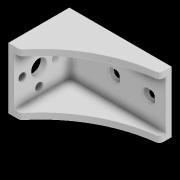
# Autodesk Inventor part: sujetador del motor
Saved by Autodesk Inventor 2020 (Build 240168000, 168)
## iProperties
Created: 2021-11-22
Part Number: sujetador del motor
Material: Generic
Document SubType Name: Modeling
Designer: juan
Density: 1 g/cm^3
Appearance: Default
Author: juan
Autodesk Inventor part; units mm, degrees
ref_plane "YZ Plane" through (0, 0, 0) normal (1, 0, 0) x (0, 1, 0)
ref_plane "XZ Plane" through (0, 0, 0) normal (0, 1, 0) x (-1, 0, 0)
ref_plane "XY Plane" through (0, 0, 0) normal (0, 0, 1) x (1, 0, 0)
sketch "Sketch1" plane through (0, 0, 0) normal (0, 0, 1) x (1, 0, 0)
  line L0 (0, 0) -> (52, 0)
  line L1 (52, 0) -> (52, 31)
  line L2 (52, 31) -> (0, 31)
  line L3 (0, 31) -> (0, 0)
  line L4 (24.7, 18.5) -> (26.7, 18.5)
  line L5 (28.7, 16.5) -> (28.7, 14.5)
  line L6 (26.7, 12.5) -> (24.7, 12.5)
  line L7 (22.7, 14.5) -> (22.7, 16.5)
  arc A0 (22.7, 14.5) -> (24.7, 12.5) centre (24.7, 14.5) ccw
  arc A1 (24.7, 18.5) -> (22.7, 16.5) centre (24.7, 16.5) ccw
  arc A2 (28.7, 16.5) -> (26.7, 18.5) centre (26.7, 16.5) ccw
  arc A3 (26.7, 12.5) -> (28.7, 14.5) centre (26.7, 14.5) ccw
  line L8 (42.542, 18.5) -> (44.542, 18.5)
  line L9 (46.542, 16.5) -> (46.542, 14.5)
  line L10 (44.542, 12.5) -> (42.542, 12.5)
  line L11 (40.542, 14.5) -> (40.542, 16.5)
  arc A4 (40.542, 14.5) -> (42.542, 12.5) centre (42.542, 14.5) ccw
  arc A5 (42.542, 18.5) -> (40.542, 16.5) centre (42.542, 16.5) ccw
  arc A6 (46.542, 16.5) -> (44.542, 18.5) centre (44.542, 16.5) ccw
  arc A7 (44.542, 12.5) -> (46.542, 14.5) centre (44.542, 14.5) ccw
  point P0 (28.7, 12.5)
  point P1 (28.7, 18.5)
  point P2 (22.7, 12.5)
  point P3 (22.7, 15.5)
  point P4 (0, 15.5)
  point P5 (46.542, 12.5)
  point P6 (46.542, 18.5)
  point P7 (40.542, 12.5)
  point P8 (40.542, 15.5)
  point P9 (28.7, 15.5)
  dimension "d0" = 52
  dimension "d1" = 31
  dimension "d2" = 6
  dimension "d3" = 6
  dimension "d4" = 2
  dimension "d5" = 22.7
  dimension "d6" = 6
  dimension "d7" = 6
  dimension "d8" = 2
  dimension "d9" = 5.458
  constraints: 24 end point, 16 point on circle, 16 tangent, 12 point on line, 8 centre point, 6 equal radius, 6 parallel, 4 midpoint, 3 horizontal, 3 perpendicular, 2 horizontal alignment
  measures "d0" distance of L2.end L1.end
  measures "d1" distance of L0.end L1.end
  measures "d2" distance of point (28.7, 12.5) point (22.7, 12.5)
  measures "d3" distance of point (28.7, 18.5) point (28.7, 12.5)
  measures "d4" radius of A0
  measures "d5" distance between parallel lines of L3 L7
  measures "d6" distance of point (46.542, 12.5) point (40.542, 12.5)
  measures "d7" distance of point (46.542, 18.5) point (46.542, 12.5)
  measures "d8" radius of A4
  measures "d9" distance between parallel lines of L1 L9
extrude "Extrusion1" add sketch "Sketch1" along normal blind 3
sketch "Sketch2" plane through (0, 0, 3) normal (0, 0, 1) x (1, 0, 0)
  line L0 (0, 31) -> (0, 0) construction
  line L1 (52, 31) -> (0, 31) construction
  line L2 (0, 0) -> (3, 0)
  line L3 (3, 0) -> (3, 31)
  line L4 (3, 31) -> (0, 31)
  line L5 (0, 31) -> (0, 0)
  dimension "d12" = 3
  constraints: 8 end point, 2 parallel, 1 horizontal, 1 perpendicular, 1 point on line
  measures "d12" distance of L4.end L3.end
extrude "Extrusion2" add sketch "Sketch2" along normal blind 28
fillet "Fillet1" radius 2 1 edges at (3, 15.5, 3)
sketch "Sketch4" plane through (0, 0, 0) normal (-1, 0, 0) x (0, 0, 1)
  point P0 (0, 0)
  point P1 (18.5, 15.5)
  point P2 (31, 15.5)
  dimension "d40" = 12.5
  constraints: 1 horizontal alignment
  measures "d40" distance of point (31, 15.5) point (18.5, 15.5)
hole "Hole1" at (0, 15.5, 18.5) direction (1, 0, 0) diameter 8 end through all
sketch "Sketch5" plane through (0, 0, 0) normal (-1, 0, 0) x (0, 0, 1)
  line L0 (0, 31) -> (0, 0) construction
  circle A0 centre (18.5, 15.5) radius 4 construction
  point P0 (18.5, 7)
  dimension "d28" = 8.5
  constraints: 1 vertical alignment
  measures "d28" distance of point (18.5, 7) A0.centre
hole "Hole2" at (0, 7, 18.5) direction (1, 0, 0) diameter 3.74 end through all
pattern_circular "Circular Pattern1" count 4 over 360 about axis through (68.0147, 15.5, 18.5) along (-1, 0, 0) of "Hole2"
sketch "Sketch7" plane through (3, 0, 31) normal (1, 0, 0) x (0, 0, -1)
  line L0 (0, 0) -> (31, 0)
  line L1 (31, 0) -> (31, 3)
  line L2 (31, 3) -> (0, 3)
  line L3 (0, 3) -> (0, 0)
  line L4 (0, 28) -> (31, 28)
  line L5 (31, 28) -> (31, 31)
  line L6 (31, 31) -> (0, 31)
  line L7 (0, 31) -> (0, 28)
  point P0 (31, 0)
  dimension "d41" = 3
  dimension "d42" = 3
  constraints: 16 end point, 4 parallel, 3 coincident, 2 horizontal, 2 perpendicular
  measures "d41" distance of L2.end L0.start
  measures "d42" distance of L5.end L4.end
extrude "Extrusion4" add sketch "Sketch7" along normal up to surface (49 mm away)
sketch "Sketch8" plane through (0, 0, 0) normal (0, -1, 0) x (1, 0, 0)
  line L0 (3, 31) -> (6, 31) construction
  line L1 (52, 3) -> (52, 6) construction
  arc A0 (6, 31) -> (52, 6) centre (58.6945, 73.1378) ccw
  line L2 (6, 31) -> (52, 31)
  line L3 (52, 31) -> (52, 6)
  point P0 (0, 0)
  dimension "d45" = 3
  dimension "d46" = 3
  dimension "d47" = 67.4708
  constraints: 8 end point, 2 horizontal, 2 point on circle, 1 centre point, 1 perpendicular, 1 vertical
  measures "d45" distance of L0.start L0.end
  measures "d46" distance of L1.start L1.end
  measures "d47" radius of A0
extrude "Extrusion5" cut sketch "Sketch8" against normal up to surface (31 mm away)
fillet "Fillet2" radius 2 2 edges at (52, 1.5, 6) (52, 29.5, 6)
body "Solid1"
